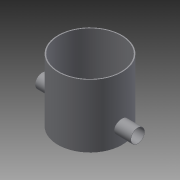
# Autodesk Inventor part: Detection Region Vacuum Collar
Saved by Autodesk Inventor 2014 (Build 180170000, 170)
## iProperties
Created: 2014-05-16
Part Number: Detection Region Vacuum Collar
Material: Generic
Document SubType Name: Modeling
Designer: ijs09
Density: 1 g/cm^3
Appearance: Default
GlobalPropertyList: <PropertyList/>
Author: ijs09
Autodesk Inventor part; units mm, degrees
ref_plane "XZ Plane" through (0, 0, 0) normal (0, 1, 0) x (-1, 0, 0)
ref_plane "XY Plane" through (0, 0, 0) normal (0, 0, 1) x (1, 0, 0)
sketch "Sketch1" plane through (0, 0, 0) normal (0, 0, 1) x (1, 0, 0)
  circle A0 centre (0, 0) radius 98.552
  circle A1 centre (0, 0) radius 101.85
  dimension "d0" = 197.104
  dimension "d1" = 203.7
  constraints: 2 centre point, 2 coincident
  measures "d0" diameter of A0
  measures "d1" diameter of A1
extrude "Extrusion1" add sketch "Sketch1" along normal blind 200
ref_plane "Work Plane1" through (101.85, 0, 0) normal (1, 0, 0) x (0, 1, 0)
sketch "Sketch3" plane through (101.85, 0, 0) normal (1, 0, 0) x (0, 1, 0)
  line L0 (-101.85, 0) -> (101.85, 0) construction
  line L1 (101.85, 200) -> (-101.85, 200) construction
  line L2 (-101.85, 0) -> (101.85, 0) projected
  line L3 (101.85, 200) -> (-101.85, 200) projected
  line L4 (101.85, 0) -> (101.85, 200) construction
  line L5 (-101.85, 0) -> (-101.85, 200) construction
  circle A0 centre (0, 50) radius 22.25
  line L6 (0, 0) -> (0, 200) construction
  dimension "d4" = 0
  dimension "d5" = 50
  dimension "d6" = 44.5
  constraints: 2 end point, 2 perpendicular, 1 centre point, 1 midpoint
  measures "d4" distance from line of L6 A0.centre
  measures "d5" distance from line of A0.centre L0
  measures "d6" diameter of A0
extrude "Extrusion2" add sketch "Sketch3" along normal blind 49.7
sketch "Sketch4" plane through (101.85, 0, 0) normal (1, 0, 0) x (0, 1, 0)
  circle A0 centre (0, 50) radius 22.25
  line L0 (0, 0) -> (0, 200) construction
  dimension "d9" = 0
  dimension "d11" = 44.5
  constraints: 2 end point, 1 centre point
  measures "d9" distance from line of L0 A0.centre
  measures "d11" diameter of A0
extrude "Extrusion3" add sketch "Sketch4" against normal up to next
ref_plane "Work Plane2" through (-101.85, 0, 0) normal (1, 0, 0) x (0, 1, 0)
sketch "Sketch6" plane through (-101.85, 0, 0) normal (1, 0, 0) x (0, 1, 0)
  circle A0 centre (0, 50) radius 22.25
  line L0 (0, 0) -> (0, 200) construction
  dimension "d16" = 0
  dimension "d18" = 44.5
  constraints: 2 end point, 1 centre point
  measures "d16" distance from line of L0 A0.centre
  measures "d18" diameter of A0
extrude "Extrusion5" add sketch "Sketch6" against normal blind 49.7
sketch "Sketch7" plane through (-101.85, 0, 0) normal (1, 0, 0) x (0, 1, 0)
  circle A0 centre (0, 50) radius 22.25
  line L0 (0, 0) -> (0, 200) construction
  dimension "d21" = 0
  dimension "d23" = 44.5
  constraints: 2 end point, 1 centre point
  measures "d21" distance from line of L0 A0.centre
  measures "d23" diameter of A0
extrude "Extrusion6" add sketch "Sketch7" along normal up to next
hole "Hole1" at (-151.55, 0, 50) direction (1, 0, 0) diameter 42.5 end through all
equation "\"d11\" = d6"
equation "\"d18\" = d6"
equation "\"d23\" = d6"
body "Solid1"
